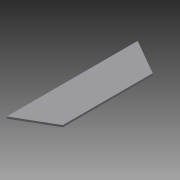
# Autodesk Inventor part: Triangle End
Saved by Autodesk Inventor 2015 (Build 190159000, 159)
## iProperties
Created: 2016-03-22
Part Number: Triangle End
Material: Generic
Document SubType Name: Modeling
Designer: Mac
Density: 1 g/cm^3
Appearance: Default
Author: Mac
Autodesk Inventor part; units mm, degrees
ref_plane "YZ Plane" through (0, 0, 0) normal (1, 0, 0) x (0, 1, 0)
ref_plane "XZ Plane" through (0, 0, 0) normal (0, 1, 0) x (-1, 0, 0)
ref_plane "XY Plane" through (0, 0, 0) normal (0, 0, 1) x (1, 0, 0)
sketch "Sketch1" plane through (0, 0, 0) normal (0, 1, 0) x (-1, 0, 0)
  line L0 (4.1559, 203.2) -> (4.1559, -203.2)
  line L1 (4.1559, -203.2) -> (156.5559, -291.1882)
  line L2 (4.1559, 203.2) -> (156.5559, 291.1882)
  line L3 (4.1559, 203.2) -> (180.1322, 203.2) construction
  line L4 (156.5559, 291.1882) -> (156.5559, -291.1882)
  point P0 (0, 0)
  point P1 (4.1559, 0)
  dimension "d0" = 120
  dimension "d1" = 30
  dimension "d2" = 406.4
  dimension "d5" = 152.4
  constraints: 10 end point, 2 vertical, 1 equal length, 1 horizontal, 1 horizontal alignment, 1 midpoint
  measures "d0" angle of L1 L0
  measures "d1" angle of L3 L2
  measures "d2" distance of L0.start L0.end
  measures "d5" distance between parallel lines of L0 L4
extrude "Extrusion1" add sketch "Sketch1" along normal blind 6.35
body "Solid1"
